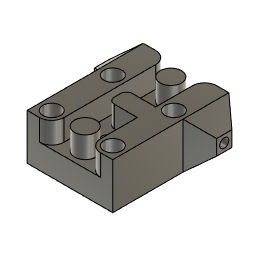
railDelta v3 (Autodesk Fusion 360 design; units mm, degrees)
Autodesk Fusion 360 part; units mm, degrees
sketch "Sketch4" plane through (0, 0, 0) normal (0, 0, 1) x (1, 0, 0)
  line L0 (7.0439, 3.6614) -> (35.0439, 3.6614)
  line L1 (35.0439, 3.6614) -> (35.0439, 41.6614)
  line L2 (35.0439, 41.6614) -> (7.0439, 41.6614)
  line L3 (7.0439, 41.6614) -> (7.0439, 3.6614)
  line L4 (15.1049, 41.6614) -> (15.1049, 3.6614)
  line L5 (27.1049, 41.6614) -> (27.1049, 3.6614)
  circle A0 centre (21.0439, 8.6614) radius 3.5
  circle A1 centre (21.0439, 15.6614) radius 1.5
  circle A2 centre (21.0439, 36.6614) radius 3.5
  circle A3 centre (21.0439, 29.6614) radius 1.5
  line L6 (27.1049, 25.6614) -> (19.5439, 25.6614)
  line L7 (17.5439, 23.6614) -> (17.5439, 21.6614)
  line L8 (19.5439, 19.6614) -> (27.1049, 19.6614)
  arc A4 (19.5439, 25.6614) -> (17.5439, 23.6614) centre (19.5439, 23.6614) ccw
  arc A5 (17.5439, 21.6614) -> (19.5439, 19.6614) centre (19.5439, 21.6614) ccw
  line L9 (11.079, 3.6614) -> (11.079, 10.1614) construction
  dimension "d17" = 28
  dimension "d18" = 38
  dimension "d24" = 7
  dimension "d28" = 3
  dimension "d30" = 7
  dimension "d31" = 7
  dimension "d32" = 3
  dimension "d41" = 2
  dimension "d42" = 2
  dimension "d55" = 6.5
  constraint horizontal L0
  constraint vertical L1
  constraint horizontal L2
  constraint vertical L3
  constraint coincident L2 L4.start
  constraint coincident L0 L4.end
  constraint perpendicular L0 L4
  constraint coincident L2 L5.start
  constraint coincident L0 L5.end
  constraint perpendicular L0 L5
  constraint coincident L5 L6.start
  constraint perpendicular L6 L7
  constraint coincident L5 L8.end
  constraint perpendicular L5 L8
  constraint tangent L6 A4
  constraint tangent L7 A4
  constraint tangent L8 A5
  constraint tangent L7 A5
  constraint coincident L0 L9.start
  constraint perpendicular L0 L9
  measures "d17" distance of L0.start L0.end
  measures "d18" distance of L0.start L2.end
  measures "d24" diameter of A0
  measures "d28" diameter of A1
  measures "d30" distance of A2.centre A3.centre
  measures "d31" diameter of A2
  measures "d32" diameter of A3
  measures "d41" radius of A4
  measures "d42" radius of A5
  measures "d55" distance of L9.start L9.end
extrude "Extrude4" add sketch "Sketch4" along normal blind 8 contours L0 L2 L4 L5 L6 L7 L8 A4 A5
extrude "Extrude5" add sketch "Sketch4" along normal blind 15 contours L0 L2 L3 L4
extrude "Extrude6" add sketch "Sketch4" along normal blind 15 contours L0 L1 L2 L5
extrude "Extrude7" add sketch "Sketch4" along normal blind 15 contours L5 L6 L7 L8 A4 A5
extrude "Extrude8" add sketch "Sketch4" along normal blind 15 contours A0
extrude "Extrude9" add sketch "Sketch4" along normal blind 15 contours A2
hole "Hole1" at (11.0744, 7.6614, 15) at (11.0744, 27.6614, 15) at (31.0744, 27.6614, 15) at (31.0744, 7.6614, 15) direction (0, 0, -1) diameter 3 end through all counterbore diameter 5.8 counterbore depth 10
sketch "Sketch16" plane through (35.0439, 0, 0) normal (1, 0, 0) x (0, 1, 0)
  line L0 (3.6614, 0) -> (41.6614, 0)
  line L1 (41.6614, 0) -> (41.6614, 15)
  line L2 (41.6614, 15) -> (3.6614, 15)
  line L3 (3.6614, 15) -> (3.6614, 0)
  line L4 (26.6614, 15) -> (26.6614, 0)
  constraint coincident L2 L4.start
  constraint coincident L0 L4.end
  constraint perpendicular L0 L4
extrude "Extrude13" add sketch "Sketch16" along normal blind 6 contours L0 L1 L2 L4
hole "Hole3" at (41.0439, 34.1614, 7.5) direction (-1, 0, 0) diameter 3 depth 12 tip angle 180
sketch "Sketch17" plane through (7.0439, 0, 0) normal (-1, 0, 0) x (0, -1, 0)
  line L0 (-41.6614, 0) -> (-3.6614, 0)
  line L1 (-3.6614, 0) -> (-3.6614, 15)
  line L2 (-3.6614, 15) -> (-41.6614, 15)
  line L3 (-41.6614, 15) -> (-41.6614, 0)
  line L4 (-26.6614, 15) -> (-26.6614, 0)
  constraint coincident L2 L4.start
  constraint coincident L0 L4.end
  constraint perpendicular L0 L4
extrude "Extrude14" add sketch "Sketch17" along normal blind 6 contours L0 L2 L3 L4
hole "Hole4" at (1.0439, 34.1614, 7.5) direction (1, 0, 0) diameter 3 depth 12 tip angle 180
sketch "Sketch19" plane through (0, 0, 0) normal (0, 0, -1) x (1, 0, 0)
  circle A0 centre (31.0744, -27.6614) radius 1.5
  circle A1 centre (11.0744, -7.6614) radius 1.5
  circle A2 centre (11.0744, -27.6614) radius 1.5
  circle A3 centre (31.0744, -7.6614) radius 1.5
  circle A4 centre (21.0439, -29.6614) radius 1.5
  circle A5 centre (21.0439, -15.6614) radius 1.5
  line L0 (1.0439, -41.6614) -> (41.0439, -41.6614)
  line L1 (41.0439, -41.6614) -> (41.0439, -26.6614)
  line L2 (41.0439, -26.6614) -> (35.0439, -26.6614)
  line L3 (35.0439, -26.6614) -> (35.0439, -3.6614)
  line L4 (35.0439, -3.6614) -> (7.0439, -3.6614)
  line L5 (7.0439, -3.6614) -> (7.0439, -26.6614)
  line L6 (7.0439, -26.6614) -> (1.0439, -26.6614)
  line L7 (1.0439, -26.6614) -> (1.0439, -41.6614)
  line L8 (1.0439, -34.1614, -7.5) -> (1.0439, -34.1614, 0) construction
  line L9 (1.0439, -34.1614) -> (41.0439, -34.1614) construction
  line L10 (41.0439, -34.1614, 0) -> (41.0439, -34.1614, -7.5) construction
  line L11 (7.0439, -26.6614) -> (7.0439, -41.6614) construction
  line L12 (35.0439, -26.6614) -> (35.0439, -41.6614) construction
  line L13 (8.2439, -31.4114) -> (5.8439, -31.4114)
  line L14 (5.8439, -31.4114) -> (5.8439, -36.9114)
  line L15 (5.8439, -36.9114) -> (8.2439, -36.9114)
  line L16 (8.2439, -36.9114) -> (8.2439, -31.4114)
  line L17 (8.2439, -31.4114) -> (5.8439, -36.9114) construction
  line L18 (5.8439, -31.4114) -> (8.2439, -36.9114) construction
  line L19 (33.8439, -31.4114) -> (36.2439, -31.4114)
  line L20 (36.2439, -31.4114) -> (36.2439, -36.9114)
  line L21 (36.2439, -36.9114) -> (33.8439, -36.9114)
  line L22 (33.8439, -36.9114) -> (33.8439, -31.4114)
  line L23 (33.8439, -31.4114) -> (36.2439, -36.9114) construction
  line L24 (36.2439, -31.4114) -> (33.8439, -36.9114) construction
  point P0 (7.0439, -34.1614)
  point P1 (35.0439, -34.1614)
  dimension "d109" = 2.4
  dimension "d110" = 5.5
  dimension "d111" = 2.4
  dimension "d112" = 5.5
  constraint midpoint L7 L9.start
  constraint midpoint L1 L9.end
  constraint coincident L5.end L6.start
  constraint coincident L0 L11.end
  constraint perpendicular L0 L11
  constraint coincident L2.end L3.start
  constraint coincident L0 L12.end
  constraint perpendicular L0 L12
  constraint horizontal L13
  constraint perpendicular L13 L14
  constraint parallel L13 L15
  constraint parallel L14 L16
  constraint coincident L17 P0
  constraint coincident L18 P0
  constraint midpoint L11 P0
  constraint horizontal L19
  constraint perpendicular L19 L20
  constraint parallel L19 L21
  constraint parallel L20 L22
  constraint coincident L23 P1
  constraint coincident L24 P1
  constraint midpoint L12 P1
  measures "d109" distance of L14.end L15.end
  measures "d110" distance of L13.end L14.end
  measures "d111" distance of L20.end L21.end
  measures "d112" distance of L19.end L20.end
extrude "Extrude15" cut sketch "Sketch19" against normal blind 10 contours L13 L14 L15 L16 | L19 L20 L21 L22
chamfer "Chamfer4" distance 5 distance2 6 4 edges at (1.0439, 26.6614, 7.5) (1.0439, 34.1614, 15) (1.0439, 41.6614, 7.5) (1.0439, 34.1614, 0) measured on face at (1.0439, 39.6601, 7.4626) measured on face at (1.0439, 39.6601, 7.4626) measured on face at (1.0439, 39.6601, 7.4626) measured on face at (1.0439, 39.6601, 7.4626)
chamfer "Chamfer5" distance 5 distance2 6 4 edges at (41.0439, 26.6614, 7.5) (41.0439, 34.1614, 15) (41.0439, 41.6614, 7.5) (41.0439, 34.1614, 0) measured on face at (41.0439, 39.6601, 7.5374) measured on face at (41.0439, 39.6601, 7.5374) measured on face at (41.0439, 39.6601, 7.5374) measured on face at (41.0439, 39.6601, 7.5374)
fillet "Fillet6" radius 4 4 edges at (15.1049, 3.6614, 11.5) (27.1049, 3.6614, 11.5) (15.1049, 41.6614, 11.5) (27.1049, 41.6614, 11.5)
